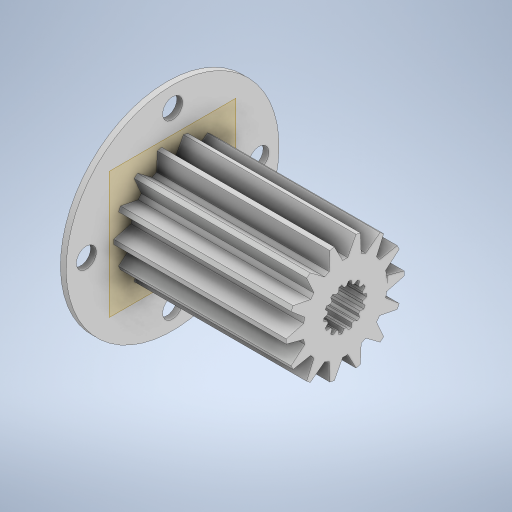
# Autodesk Inventor part: MotorAdapter
Saved by Autodesk Inventor 2023 (Build 270158000, 158)
## iProperties
Created: 2023-02-23
Part Number: MotorAdapter
Material: Generic
Document SubType Name: Sheet Metal
Designer: Charles Kelly
Density: 1 g/cm^3
Sheet Metal Rule: Default_mm
Appearance: Default
Author: Charles Kelly
Autodesk Inventor part; units mm, degrees
ref_plane "YZ Plane" through (0, 0, 0) normal (1, 0, 0) x (0, 1, 0)
ref_plane "XZ Plane" through (0, 0, 0) normal (0, 1, 0) x (-1, 0, 0)
ref_plane "XY Plane" through (0, 0, 0) normal (0, 0, 1) x (1, 0, 0)
sketch "Sketch1" plane through (0, 0, 0) normal (1, 0, 0) x (0, 1, 0)
  circle A0 centre (-3.2599, 0) radius 15
  circle A1 centre (-3.2599, -15) radius 1.75
  circle A2 centre (11.7401, 0) radius 1.75
  circle A3 centre (-3.2599, 15) radius 1.75
  circle A4 centre (-18.2599, 0) radius 1.75
  circle A5 centre (-3.2599, 0) radius 18.5
  circle A6 centre (-3.2599, 0) radius 1.75
  point P0 (0, 0)
  dimension "d0" = 30
  dimension "d1" = 3.5
  dimension "d4" = 360
  dimension "d6" = 37
  dimension "d25" = 3.5
  constraints: 6 centre point, 2 coincident, 1 vertical alignment, 11 other
  measures "d1" diameter of A1
  measures "d6" diameter of A5
  measures "d25" diameter of A6
ref_plane "Work Plane1" through (1, -3.2599, 0) normal (1, 0, 0) x (0, 0, -1)
sketch "Sketch2" plane through (1, -3.2599, 0) normal (1, 0, 0) x (0, 0, -1)
  circle A0 centre (0, 0) radius 3.1115
  line L0 (0.1996, 3.1051) -> (0.5779, 3.676)
  line L1 (0.5779, 3.676) -> (1.0739, 3.5637)
  line L2 (1.0739, 3.5637) -> (1.1674, 2.8842)
  line L3 (-1.1674, 2.8842) -> (-1.0743, 3.5626)
  line L4 (-1.0743, 3.5626) -> (-0.5787, 3.6768)
  line L5 (-0.5787, 3.6768) -> (-0.1996, 3.1051)
  line L6 (-2.3032, 2.092) -> (-2.5137, 2.7437)
  line L7 (-2.5137, 2.7437) -> (-2.1167, 3.0616)
  line L8 (-2.1167, 3.0616) -> (-1.5271, 2.711)
  line L9 (-2.9828, 0.8855) -> (-3.4552, 1.3813)
  line L10 (-3.4552, 1.3813) -> (-3.2354, 1.84)
  line L11 (-3.2354, 1.84) -> (-2.5521, 1.78)
  line L12 (-3.0717, -0.4964) -> (-3.7124, -0.2546)
  line L13 (-3.7124, -0.2546) -> (-3.7134, 0.254)
  line L14 (-3.7134, 0.254) -> (-3.0717, 0.4964)
  line L15 (-2.5521, -1.78) -> (-3.2343, -1.8401)
  line L16 (-3.2343, -1.8401) -> (-3.4558, -1.3823)
  line L17 (-3.4558, -1.3823) -> (-2.9828, -0.8855)
  line L18 (-1.5271, -2.711) -> (-2.1156, -3.0612)
  line L19 (-2.1156, -3.0612) -> (-2.5138, -2.7449)
  line L20 (-2.5138, -2.7449) -> (-2.3032, -2.092)
  line L21 (-0.1996, -3.1051) -> (-0.5779, -3.676)
  line L22 (-0.5779, -3.676) -> (-1.0739, -3.5637)
  line L23 (-1.0739, -3.5637) -> (-1.1674, -2.8842)
  line L24 (1.1674, -2.8842) -> (1.0743, -3.5626)
  line L25 (1.0743, -3.5626) -> (0.5787, -3.6768)
  line L26 (0.5787, -3.6768) -> (0.1996, -3.1051)
  line L27 (2.3032, -2.092) -> (2.5137, -2.7437)
  line L28 (2.5137, -2.7437) -> (2.1167, -3.0616)
  line L29 (2.1167, -3.0616) -> (1.5271, -2.711)
  line L30 (2.9828, -0.8855) -> (3.4552, -1.3813)
  line L31 (3.4552, -1.3813) -> (3.2354, -1.84)
  line L32 (3.2354, -1.84) -> (2.5521, -1.78)
  line L33 (3.0717, 0.4964) -> (3.7124, 0.2546)
  line L34 (3.7124, 0.2546) -> (3.7134, -0.254)
  line L35 (3.7134, -0.254) -> (3.0717, -0.4964)
  line L36 (2.5521, 1.78) -> (3.2343, 1.8401)
  line L37 (3.2343, 1.8401) -> (3.4558, 1.3823)
  line L38 (3.4558, 1.3823) -> (2.9828, 0.8855)
  line L39 (1.5271, 2.711) -> (2.1156, 3.0612)
  line L40 (2.1156, 3.0612) -> (2.5138, 2.7449)
  line L41 (2.5138, 2.7449) -> (2.3032, 2.092)
  point P0 (3.0717, 0.4964)
  point P1 (-3.0717, 0.4964)
  point P2 (-3.0717, -0.4964)
  point P3 (-2.9828, -0.8855)
  point P4 (-2.5521, -1.78)
  point P5 (-1.5271, -2.711)
  point P6 (-1.1674, -2.8842)
  point P7 (0.1996, -3.1051)
  point P8 (2.3032, -2.092)
  point P9 (2.9828, -0.8855)
  dimension "d11" = 360
  constraints: 84 end point, 1 coincident, 101 other
ref_plane "Work Plane2" through (1, -3.2599, 0) normal (1, 0, 0) x (0, 0, -1)
sketch "Sketch3" plane through (1, -3.2599, 0) normal (1, 0, 0) x (0, 0, -1)
  circle A0 centre (0, 0) radius 7.3152
  line L0 (7.3152, 0) -> (7.3152, 1.168)
  line L1 (7.3152, 1.168) -> (10.2374, 0.3954)
  line L2 (7.3152, 1.168) -> (10.3378, 1.168) construction
  line L3 (10.2374, 0.3954) -> (10.2374, 0)
  line L4 (7.3152, 1.168) -> (7.2171, 1.1939)
  line L5 (10.2374, 0) -> (9.5494, 0)
  line L6 (7.3152, -1.168) -> (10.2374, -0.3954)
  line L7 (10.2374, -0.3954) -> (10.2374, 0)
  line L8 (7.3152, -1.168) -> (7.2171, -1.1939)
  line L9 (7.0975, 2.1216) -> (7.0204, 2.0557)
  line L10 (7.0975, 2.1216) -> (9.3951, 4.0856)
  line L11 (9.3951, 4.0856) -> (9.2236, 4.4418)
  line L12 (9.052, 4.7981) -> (9.2236, 4.4418)
  line L13 (6.084, 4.2263) -> (9.052, 4.7981)
  line L14 (6.084, 4.2263) -> (5.9844, 4.2071)
  line L15 (5.4741, 4.991) -> (5.4333, 4.8982)
  line L16 (5.4741, 4.991) -> (6.692, 7.7574)
  line L17 (6.692, 7.7574) -> (6.3829, 8.0039)
  line L18 (6.0738, 8.2504) -> (6.3829, 8.0039)
  line L19 (3.6478, 6.4475) -> (6.0738, 8.2504)
  line L20 (3.6478, 6.4475) -> (3.5663, 6.387)
  line L21 (2.7665, 6.8719) -> (2.77, 6.7705)
  line L22 (2.7665, 6.8719) -> (2.6635, 9.8927)
  line L23 (2.6635, 9.8927) -> (2.278, 9.9807)
  line L24 (1.8926, 10.0687) -> (2.278, 9.9807)
  line L25 (0.4891, 7.3917) -> (1.8926, 10.0687)
  line L26 (0.4891, 7.3917) -> (0.442, 7.3018)
  line L27 (-0.4891, 7.3917) -> (-0.442, 7.3018)
  line L28 (-0.4891, 7.3917) -> (-1.8926, 10.0687)
  line L29 (-1.8926, 10.0687) -> (-2.278, 9.9807)
  line L30 (-2.6635, 9.8927) -> (-2.278, 9.9807)
  line L31 (-2.7665, 6.8719) -> (-2.6635, 9.8927)
  line L32 (-2.7665, 6.8719) -> (-2.77, 6.7705)
  line L33 (-3.6478, 6.4475) -> (-3.5663, 6.387)
  line L34 (-3.6478, 6.4475) -> (-6.0738, 8.2504)
  line L35 (-6.0738, 8.2504) -> (-6.3829, 8.0039)
  line L36 (-6.692, 7.7574) -> (-6.3829, 8.0039)
  line L37 (-5.4741, 4.991) -> (-6.692, 7.7574)
  line L38 (-5.4741, 4.991) -> (-5.4333, 4.8982)
  line L39 (-6.084, 4.2263) -> (-5.9844, 4.2071)
  line L40 (-6.084, 4.2263) -> (-9.052, 4.7981)
  line L41 (-9.052, 4.7981) -> (-9.2236, 4.4418)
  line L42 (-9.3951, 4.0856) -> (-9.2236, 4.4418)
  line L43 (-7.0975, 2.1216) -> (-9.3951, 4.0856)
  line L44 (-7.0975, 2.1216) -> (-7.0204, 2.0557)
  line L45 (-7.3152, 1.168) -> (-7.2171, 1.1939)
  line L46 (-7.3152, 1.168) -> (-10.2374, 0.3954)
  line L47 (-10.2374, 0.3954) -> (-10.2374, 0)
  line L48 (-10.2374, -0.3954) -> (-10.2374, 0)
  line L49 (-7.3152, -1.168) -> (-10.2374, -0.3954)
  line L50 (-7.3152, -1.168) -> (-7.2171, -1.1939)
  line L51 (-7.0975, -2.1216) -> (-7.0204, -2.0557)
  line L52 (-7.0975, -2.1216) -> (-9.3951, -4.0856)
  line L53 (-9.3951, -4.0856) -> (-9.2236, -4.4418)
  line L54 (-9.052, -4.7981) -> (-9.2236, -4.4418)
  line L55 (-6.084, -4.2263) -> (-9.052, -4.7981)
  line L56 (-6.084, -4.2263) -> (-5.9844, -4.2071)
  line L57 (-5.4741, -4.991) -> (-5.4333, -4.8982)
  line L58 (-5.4741, -4.991) -> (-6.692, -7.7574)
  line L59 (-6.692, -7.7574) -> (-6.3829, -8.0039)
  line L60 (-6.0738, -8.2504) -> (-6.3829, -8.0039)
  line L61 (-3.6478, -6.4475) -> (-6.0738, -8.2504)
  line L62 (-3.6478, -6.4475) -> (-3.5663, -6.387)
  line L63 (-2.7665, -6.8719) -> (-2.77, -6.7705)
  line L64 (-2.7665, -6.8719) -> (-2.6635, -9.8927)
  line L65 (-2.6635, -9.8927) -> (-2.278, -9.9807)
  line L66 (-1.8926, -10.0687) -> (-2.278, -9.9807)
  line L67 (-0.4891, -7.3917) -> (-1.8926, -10.0687)
  line L68 (-0.4891, -7.3917) -> (-0.442, -7.3018)
  line L69 (0.4891, -7.3917) -> (0.442, -7.3018)
  line L70 (0.4891, -7.3917) -> (1.8926, -10.0687)
  line L71 (1.8926, -10.0687) -> (2.278, -9.9807)
  line L72 (2.6635, -9.8927) -> (2.278, -9.9807)
  line L73 (2.7665, -6.8719) -> (2.6635, -9.8927)
  line L74 (2.7665, -6.8719) -> (2.77, -6.7705)
  line L75 (3.6478, -6.4475) -> (3.5663, -6.387)
  line L76 (3.6478, -6.4475) -> (6.0738, -8.2504)
  line L77 (6.0738, -8.2504) -> (6.3829, -8.0039)
  line L78 (6.692, -7.7574) -> (6.3829, -8.0039)
  line L79 (5.4741, -4.991) -> (6.692, -7.7574)
  line L80 (5.4741, -4.991) -> (5.4333, -4.8982)
  line L81 (6.084, -4.2263) -> (5.9844, -4.2071)
  line L82 (6.084, -4.2263) -> (9.052, -4.7981)
  line L83 (9.052, -4.7981) -> (9.2236, -4.4418)
  line L84 (9.3951, -4.0856) -> (9.2236, -4.4418)
  line L85 (7.0975, -2.1216) -> (9.3951, -4.0856)
  line L86 (7.0975, -2.1216) -> (7.0204, -2.0557)
  point P0 (0, 3.2599)
  point P1 (-7.2171, 1.1939)
  point P2 (-7.2171, -1.1939)
  point P3 (-7.0204, -2.0557)
  point P4 (-5.9844, -4.2071)
  point P5 (5.4333, -4.8982)
  point P6 (7.0204, -2.0557)
  dimension "d12" = 14.6304
  dimension "d14" = 1.168
  dimension "d15" = 3.0226
  dimension "d16" = 14.81
  dimension "d19" = 360
  constraints: 174 end point, 28 point on line, 3 symmetric about line, 3 vertical, 2 horizontal, 1 equal length, 187 other
  measures "d14" distance of L0.start L0.end
  measures "d15" distance of L0.end L1.end
  measures "d16" angle of L1 L2
extrude "Extrusion2" add sketch "Sketch3" along normal blind 30 contours A0 | L0 L1 L3 L7 L6 L8 A0 | A0 L14 L13 L12 L11 L10 L9 | L86 L85 L84 L83 L82 L81 A0 | A0 L20 L19 L18 L17 L16 L15 | L80 L79 L78 L77 L76 L75 A0 | A0 L26 L25 L24 L23 L22 L21 | L74 L73 L72 L71 L70 L69 A0 | A0 L32 L31 L30 L29 L28 L27 | L68 L67 L66 L65 L64 L63 A0 | A0 L38 L37 L36 L35 L34 L33 | L62 L61 L60 L59 L58 L57 A0 | A0 L44 L43 L42 L41 L40 L39 | L56 L55 L54 L53 L52 L51 A0 | A0 L50 L49 L48 L47 L46 L45
extrude "Extrusion3" cut sketch "Sketch2" along normal blind 30
extrude "Extrusion4" add sketch "Sketch1" along normal blind 1 contours A2 A0 A1 A4 A3 | A5
equation "\"GapSize\" = Thickness"
equation "\"BendRadius\" = Thickness"
equation "\"MinimumRemnant\" = 2 * Thickness"
equation "\"BendReliefDepth\" = 0.5 * Thickness"
equation "\"BendReliefWidth\" = Thickness"
equation "\"CornerReliefSize\" = 4 * Thickness"
equation "\"JacobiRadiusSize\" = BendRadius"
equation "\"TransitionRadius\" = BendRadius"
equation "\"Thickness\" = 0.5"
body "Solid1"
